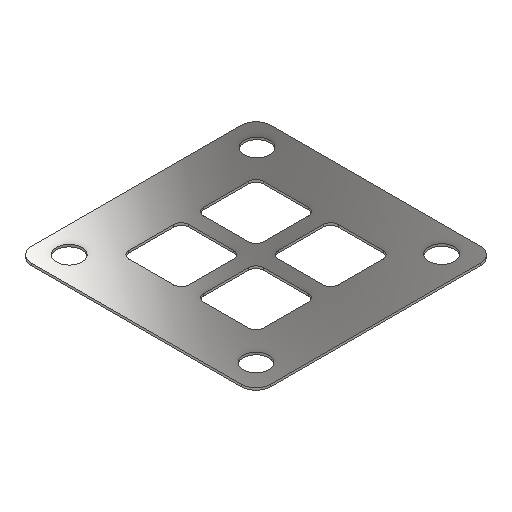
# Autodesk Inventor part: B_holder_up_muti-holes
Saved by Autodesk Inventor 2026.2 (Build 302298000, 298)
## iProperties
Created: 2026-02-20
Part Number: B_holder_up_muti-holes
Material: ステンレス鋼 440C
Document SubType Name: Modeling
Designer: zetsu
Density: 7.75 g/cm^3
Appearance: 半つや出し
Author: zetsu
Autodesk Inventor part; units mm, degrees
ref_plane "YZ Plane" through (0, 0, 0) normal (1, 0, 0) x (0, 1, 0)
ref_plane "XZ Plane" through (0, 0, 0) normal (0, 1, 0) x (-1, 0, 0)
ref_plane "XY Plane" through (0, 0, 0) normal (0, 0, 1) x (1, 0, 0)
sketch "スケッチ1" plane through (0, 0, 0) normal (0, 1, 0) x (-1, 0, 0)
  line L0 (16, -16) -> (16, 16)
  line L1 (16, 16) -> (-16, 16)
  line L2 (-16, 16) -> (-16, -16)
  line L3 (-16, -16) -> (16, -16)
  line L4 (0, 0) -> (0, -32.6995) construction
  line L5 (0, 0) -> (-21.9909, 0) construction
  point P0 (0, 16)
  dimension "d0" = 32
  dimension "d1" = 32
  constraints: 12 end point, 3 perpendicular, 2 vertical, 1 horizontal, 1 midpoint, 2 other
  measures "d0" distance of L0.end L0.start
  measures "d1" distance of L1.end L0.end
extrude "押し出し1" add sketch "スケッチ1" along normal blind 0.3
sketch "スケッチ7" plane through (0, 0.3, 0) normal (0, 1, 0) x (1, 0, 0)
  circle A0 centre (-12.5, -12.5) radius 1.7
  circle A1 centre (12.5, -12.5) radius 1.7
  circle A2 centre (12.3554, 12.5) radius 1.7
  circle A3 centre (-12.3554, 12.5) radius 1.7
  line L0 (0, 0) -> (0, 34.4459) construction
  point P0 (-16, -16)
  dimension "d47" = 3.4
  dimension "d48" = 3.4
  dimension "d49" = 3.4
  dimension "d50" = 3.4
  dimension "d51" = 25
  dimension "d52" = 25
  dimension "d55" = 3.5
  constraints: 4 centre point, 2 end point, 2 symmetric about line, 1 vertical
  measures "d47" diameter of A0
  measures "d48" diameter of A1
  measures "d49" diameter of A2
  measures "d50" diameter of A3
  measures "d51" distance of A1.centre A0.centre
  measures "d52" vertical distance of A1.centre A2.centre
  measures "d55" horizontal distance of point (-16, -16) A0.centre
extrude "押し出し6" cut sketch "スケッチ7" against normal through all
sketch "スケッチ10" plane through (0, 0.3, 0) normal (0, 1, 0) x (1, 0, 0)
  line L0 (-1, 1) -> (-9, 1)
  line L1 (-9, 1) -> (-9, 9)
  line L2 (-9, 9) -> (-1, 9)
  line L3 (-1, 9) -> (-1, 1)
  line L4 (-9, -1) -> (-1, -1)
  line L5 (-9, -9) -> (-9, -1)
  line L6 (-1, -9) -> (-9, -9)
  line L7 (-1, -1) -> (-1, -9)
  line L8 (1, -9) -> (1, -1)
  line L9 (9, -9) -> (1, -9)
  line L10 (9, -1) -> (9, -9)
  line L11 (1, -1) -> (9, -1)
  line L12 (9, 1) -> (1, 1)
  line L13 (9, 9) -> (9, 1)
  line L14 (1, 9) -> (9, 9)
  line L15 (1, 1) -> (1, 9)
  point P0 (0, 0)
  dimension "d71" = 8
  dimension "d72" = 8
  dimension "d73" = 1
  dimension "d74" = 1
  dimension "d77" = 360
  constraints: 32 end point, 2 parallel, 1 horizontal, 1 perpendicular, 33 other
  measures "d71" distance of L1.end L2.end
  measures "d72" distance of L0.end L1.end
  measures "d73" horizontal distance of point (0, 0) L0.start
  measures "d74" horizontal distance of point (0, 0) L0.start
extrude "押し出し9" cut sketch "スケッチ10" against normal through all
fillet "フィレット1" radius 2 4 edges at (-16, 0.15, 16) (16, 0.15, 16) (16, 0.15, -16) (-16, 0.15, -16)
fillet "フィレット2" radius 1 16 edges at (-9, 0.15, -9) (-9, 0.15, -1) (-1, 0.15, -9) (-1, 0.15, -1) (-1, 0.15, 1) (1, 0.15, 1) (1, 0.15, -1) (-9, 0.15, 1) (-9, 0.15, 9) (-1, 0.15, 9) (1, 0.15, 9) (9, 0.15, 9) (9, 0.15, 1) (9, 0.15, -1) (9, 0.15, -9) (1, 0.15, -9)
